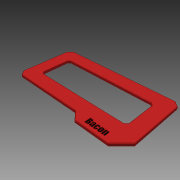
# Autodesk Inventor part: display_2004_frame
Saved by Autodesk Inventor 2014 (Build 180170000, 170)
## iProperties
Created: 2014-01-22
Part Number: display_2004_frame
Material: ABS Plastic
Document SubType Name: Modeling
Designer: buben
Density: 1.06 g/cm^3
Appearance: Light Red
Author: buben
Autodesk Inventor part; units mm, degrees
ref_plane "YZ Plane" through (0, 0, 0) normal (1, 0, 0) x (0, 1, 0)
ref_plane "XZ Plane" through (0, 0, 0) normal (0, 1, 0) x (-1, 0, 0)
ref_plane "XY Plane" through (0, 0, 0) normal (0, 0, 1) x (1, 0, 0)
sketch "Sketch1" plane through (0, 0, 0) normal (0, 1, 0) x (-1, 0, 0)
  line L0 (2, 0) -> (78, 0)
  line L1 (80, 2) -> (80, 25)
  line L2 (78, 27) -> (2, 27)
  line L3 (0, 25) -> (0, 2)
  line L4 (0, 25) -> (2, 27)
  line L5 (78, 27) -> (80, 25)
  line L6 (80, 2) -> (78, 0)
  line L7 (2, 0) -> (0, 2)
  line L8 (-8, 39) -> (88, 39)
  line L9 (92, 35) -> (92, -8)
  line L10 (88, -12) -> (-8, -12)
  line L11 (-12, -8) -> (-12, 35)
  line L12 (-12, 35) -> (-8, 39)
  line L13 (88, 39) -> (92, 35)
  line L14 (92, -8) -> (88, -12)
  line L15 (-8, -12) -> (-12, -8)
  point P0 (0, 0)
  point P1 (80, 27)
  point P2 (80, 0)
  point P3 (0, 27)
  point P4 (-12, 39)
  point P5 (92, -12)
  point P6 (92, 39)
  point P7 (-12, -12)
  point P8 (40, 39)
  point P9 (40, 27)
  point P10 (-12, 13.5)
  point P11 (0, 13.5)
  dimension "d0" = 2
  dimension "d1" = 2
  dimension "d2" = 2
  dimension "d3" = 2
  dimension "d4" = 2
  dimension "d5" = 2
  dimension "d6" = 2
  dimension "d7" = 2
  dimension "d8" = 80
  dimension "d9" = 27
  dimension "d10" = 4
  dimension "d11" = 4
  dimension "d12" = 4
  dimension "d13" = 4
  dimension "d14" = 4
  dimension "d15" = 4
  dimension "d16" = 4
  dimension "d17" = 4
  dimension "d18" = 12
  dimension "d19" = 12
  constraints: 32 end point, 16 point on line, 4 midpoint, 4 parallel, 2 horizontal, 2 perpendicular, 1 horizontal alignment, 1 vertical alignment
  measures "d0" distance of L3.start point (0, 27)
  measures "d1" distance of L2.end point (0, 27)
  measures "d2" distance of L2.start point (80, 27)
  measures "d3" distance of L1.end point (80, 27)
  measures "d4" distance of L1.start point (80, 0)
  measures "d5" distance of L0.end point (80, 0)
  measures "d6" distance of L0.start point (0, 0)
  measures "d7" distance of L3.end point (0, 0)
  measures "d8" distance between parallel lines of L1 L3
  measures "d9" distance between parallel lines of L0 L2
  measures "d10" distance of L11.end point (-12, 39)
  measures "d11" distance of L8.start point (-12, 39)
  measures "d12" distance of L8.end point (92, 39)
  measures "d13" distance of L9.start point (92, 39)
  measures "d14" distance of L9.end point (92, -12)
  measures "d15" distance of L10.start point (92, -12)
  measures "d16" distance of L10.end point (-12, -12)
  measures "d17" distance of L11.start point (-12, -12)
  measures "d18" distance between parallel lines of L3 L11
  measures "d19" distance between parallel lines of L2 L8
extrude "Extrusion1" add sketch "Sketch1" along normal blind 2
sketch "Sketch2" plane through (0, 2, 0) normal (0, 1, 0) x (1, 0, 0)
  line L0 (-92, -35) -> (-88, -39) projected
  line L1 (-88, -39) -> (8, -39) projected
  line L2 (8, -39) -> (2, -45)
  line L3 (2, -45) -> (-24, -45)
  line L4 (-24, -45) -> (-30, -39)
  point P0 (0, 0)
  dimension "d22" = 6
  dimension "d23" = 26
  constraints: 6 end point, 2 perpendicular, 1 parallel, 1 point on line
  measures "d22" distance between parallel lines of L1 L3
  measures "d23" distance of L2.end L3.end
extrude "Extrusion2" add sketch "Sketch2" against normal blind 2
chamfer "Chamfer1" distance 0.3 angle 45 18 edges at (-80, 2, 13.5) (-79, 2, 26) (-40, 2, 27) (-79, 2, 1) (-40, 2, 0) (-1, 2, 26) (0, 2, 13.5) (-1, 2, 1) (7, 2, 40) (12, 2, 13.5) (10, 2, -10) (-11, 2, 45) (-27, 2, 42) (-59, 2, 39) (-90, 2, 37) (-92, 2, 13.5) (-90, 2, -10) (-40, 2, -12)
sketch "Sketch3" plane through (0, 2, 0) normal (0, 1, 0) x (1, 0, 0)
  line L0 (-23.8757, -44.7) -> (-29.8757, -38.7) projected
  line L1 (1.8757, -44.7) -> (-23.8757, -44.7) projected
  line L2 (11.7, -34.8757) -> (1.8757, -44.7) projected
  line L3 (-29.8757, -38.7) -> (-87.8757, -38.7) projected
  line L4 (-21, -37.2) -> (-1, -37.2) construction
  line L5 (-1, -37.2) -> (-1, -42.2) construction
  line L6 (-1, -42.2) -> (-21, -42.2) construction
  line L7 (-21, -42.2) -> (-21, -37.2) construction
  line L8 (-21, -39.7) -> (-28.8757, -39.7) construction
  line L9 (-1, -39.7) -> (6.8757, -39.7) construction
  line L10 (-18.9145, -37.2) -> (-17.6183, -37.2)
  spline S0 degree 2 poles (-17.6183, -37.2) (-17.0004, -37.2) (-16.3674, -37.3922) (-15.9793, -37.9762) (-15.9793, -38.6243) knots 0 0 0 1 2 3 3 3
  spline S1 degree 2 poles (-15.9793, -38.6243) (-15.9793, -39.0613) (-16.2543, -39.408) (-16.6613, -39.4984) knots 0 0 0 1 2 2 2
  spline S2 degree 2 poles (-16.6613, -39.4984) (-16.2091, -39.6039) (-15.8888, -40.0749) (-15.8888, -40.5647) knots 0 0 0 1 2 2 2
  line L11 (-15.8888, -40.5647) -> (-15.8888, -41.0244)
  spline S3 degree 2 poles (-15.8888, -41.0244) (-15.8888, -41.5331) (-16.1187, -42.0191) (-16.6274, -42.2) (-17.4111, -42.2) knots 0 0 0 1 2 3 3 3
  line L12 (-17.4111, -42.2) -> (-18.9145, -42.2)
  line L13 (-18.9145, -42.2) -> (-18.9145, -37.2)
  line L14 (-17.6145, -39.9468) -> (-17.6145, -41.3447)
  spline S4 degree 2 poles (-17.6145, -41.3447) (-17.3395, -41.3372) (-17.1888, -41.1827) (-17.1888, -40.8775) knots 0 0 0 1 2 2 2
  line L15 (-17.1888, -40.8775) -> (-17.1888, -40.414)
  spline S5 degree 2 poles (-17.1888, -40.414) (-17.1888, -40.09) (-17.3244, -39.9543) (-17.6145, -39.9468) knots 0 0 0 1 2 2 2
  line L16 (-17.6145, -38.0553) -> (-17.6145, -39.1668)
  spline S6 degree 2 poles (-17.6145, -39.1668) (-17.5317, -39.1631) (-17.4864, -39.1631) knots 0 0 0 1 1 1
  spline S7 degree 2 poles (-17.4864, -39.1631) (-17.2943, -39.1631) (-17.1888, -38.9747) (-17.1888, -38.5301) knots 0 0 0 1 2 2 2
  spline S8 degree 2 poles (-17.1888, -38.5301) (-17.1888, -38.2965) (-17.2754, -38.1081) (-17.4148, -38.0591) (-17.6145, -38.0553) knots 0 0 0 1 2 3 3 3
  line L17 (-14.344, -39.6868) -> (-15.5158, -39.6868)
  line L18 (-15.5158, -39.6868) -> (-15.5158, -39.4118)
  spline S9 degree 2 poles (-15.5158, -39.4118) (-15.5158, -38.937) (-15.2973, -38.4208) (-14.6341, -38.0252) (-14.1066, -38.0252) knots 0 0 0 1 2 3 3 3
  spline S10 degree 2 poles (-14.1066, -38.0252) (-13.4736, -38.0252) (-12.8293, -38.4735) (-12.7012, -39.1254) (-12.7012, -40.1427) knots 0 0 0 1 2 3 3 3
  line L19 (-12.7012, -40.1427) -> (-12.7012, -42.2)
  line L20 (-12.7012, -42.2) -> (-13.9145, -42.2)
  line L21 (-13.9145, -42.2) -> (-13.9145, -41.8345)
  spline S11 degree 2 poles (-13.9145, -41.8345) (-14.0275, -42.0531) (-14.3892, -42.2754) (-14.6417, -42.2754) knots 0 0 0 1 2 2 2
  spline S12 degree 2 poles (-14.6417, -42.2754) (-14.9695, -42.2754) (-15.5158, -41.9061) (-15.5158, -41.2844) knots 0 0 0 1 2 2 2
  line L22 (-15.5158, -41.2844) -> (-15.5158, -40.9491)
  spline S13 degree 2 poles (-15.5158, -40.9491) (-15.5158, -40.4894) (-15.2257, -40.154) (-14.6492, -39.9317) knots 0 0 0 1 2 2 2
  spline S14 degree 2 poles (-14.6492, -39.9317) (-14.035, -39.6906) (-13.9484, -39.5248) (-13.9484, -39.2686) knots 0 0 0 1 2 2 2
  spline S15 degree 2 poles (-13.9484, -39.2686) (-13.9484, -38.9483) (-14.0426, -38.7524) (-14.1556, -38.7524) knots 0 0 0 1 2 2 2
  spline S16 degree 2 poles (-14.1556, -38.7524) (-14.2837, -38.7524) (-14.344, -38.9144) (-14.344, -39.2573) knots 0 0 0 1 2 2 2
  line L23 (-14.344, -39.2573) -> (-14.344, -39.6868)
  spline S17 degree 2 poles (-13.9484, -40.2482) (-14.2498, -40.4668) (-14.344, -40.7644) (-14.344, -41.0433) knots 0 0 0 1 2 2 2
  spline S18 degree 2 poles (-14.344, -41.0433) (-14.344, -41.3635) (-14.2611, -41.5482) (-14.1368, -41.5482) knots 0 0 0 1 2 2 2
  spline S19 degree 2 poles (-14.1368, -41.5482) (-14.02, -41.5482) (-13.9484, -41.4012) (-13.9484, -41.0922) knots 0 0 0 1 2 2 2
  line L24 (-13.9484, -41.0922) -> (-13.9484, -40.2482)
  line L25 (-9.5136, -39.6491) -> (-10.6891, -39.6491)
  line L26 (-10.6891, -39.6491) -> (-10.6891, -39.1744)
  spline S20 degree 2 poles (-10.6891, -39.1744) (-10.6891, -38.9295) (-10.7683, -38.7524) (-10.8775, -38.7524) knots 0 0 0 1 2 2 2
  spline S21 degree 2 poles (-10.8775, -38.7524) (-10.9868, -38.7524) (-11.0622, -38.9069) (-11.0622, -39.1744) knots 0 0 0 1 2 2 2
  line L27 (-11.0622, -39.1744) -> (-11.0622, -41.1111)
  spline S22 degree 2 poles (-11.0622, -41.1111) (-11.0622, -41.3296) (-10.9491, -41.5482) (-10.8436, -41.5482) knots 0 0 0 1 2 2 2
  spline S23 degree 2 poles (-10.8436, -41.5482) (-10.7155, -41.5482) (-10.6251, -41.3183) (-10.6251, -41.0018) knots 0 0 0 1 2 2 2
  line L28 (-10.6251, -41.0018) -> (-10.6251, -40.5157)
  line L29 (-10.6251, -40.5157) -> (-9.5136, -40.5157)
  spline S24 degree 2 poles (-9.5136, -40.5157) (-9.5173, -41.0056) (-9.5814, -41.4992) (-9.9318, -42.0116) (-10.4932, -42.2754) (-10.9077, -42.2754) knots 0 0 0 1 2 3 4 4 4
  spline S25 degree 2 poles (-10.9077, -42.2754) (-11.4352, -42.2754) (-12.0531, -41.9136) (-12.3093, -41.2618) (-12.3093, -40.6627) knots 0 0 0 1 2 3 3 3
  line L30 (-12.3093, -40.6627) -> (-12.3093, -39.4946)
  spline S26 degree 2 poles (-12.3093, -39.4946) (-12.3093, -38.9747) (-12.0983, -38.4434) (-11.4126, -38.0252) (-10.9228, -38.0252) knots 0 0 0 1 2 3 3 3
  spline S27 degree 2 poles (-10.9228, -38.0252) (-10.4329, -38.0252) (-9.7434, -38.4396) (-9.5136, -39.0689) (-9.5136, -39.6491) knots 0 0 0 1 2 3 3 3
  line L31 (-6.3222, -39.5399) -> (-6.3222, -40.5459)
  spline S28 degree 2 poles (-6.3222, -40.5459) (-6.3222, -41.096) (-6.4314, -41.6122) (-6.7969, -42.0606) (-7.3696, -42.2754) (-7.7389, -42.2754) knots 0 0 0 1 2 3 4 4 4
  spline S29 degree 2 poles (-7.7389, -42.2754) (-8.1534, -42.2754) (-8.7298, -42.0945) (-9.0463, -41.7252) (-9.182, -41.2015) (-9.182, -40.6815) knots 0 0 0 1 2 3 4 4 4
  line L32 (-9.182, -40.6815) -> (-9.182, -39.6303)
  spline S30 degree 2 poles (-9.182, -39.6303) (-9.182, -39.0576) (-8.9333, -38.4133) (-8.2928, -38.0252) (-7.7916, -38.0252) knots 0 0 0 1 2 3 3 3
  spline S31 degree 2 poles (-7.7916, -38.0252) (-7.3734, -38.0252) (-6.7705, -38.2739) (-6.4427, -38.677) (-6.3222, -39.1028) (-6.3222, -39.5399) knots 0 0 0 1 2 3 4 4 4
  spline S32 degree 2 poles (-7.5693, -39.2309) (-7.5693, -38.9144) (-7.6372, -38.7524) (-7.7502, -38.7524) knots 0 0 0 1 2 2 2
  spline S33 degree 2 poles (-7.7502, -38.7524) (-7.8595, -38.7524) (-7.9348, -38.9144) (-7.9348, -39.2309) knots 0 0 0 1 2 2 2
  line L33 (-7.9348, -39.2309) -> (-7.9348, -41.0809)
  spline S34 degree 2 poles (-7.9348, -41.0809) (-7.9348, -41.3711) (-7.8595, -41.5482) (-7.7502, -41.5482) knots 0 0 0 1 2 2 2
  spline S35 degree 2 poles (-7.7502, -41.5482) (-7.6409, -41.5482) (-7.5693, -41.3861) (-7.5693, -41.1224) knots 0 0 0 1 2 2 2
  line L34 (-7.5693, -41.1224) -> (-7.5693, -39.2309)
  line L35 (-4.6417, -38.1005) -> (-4.6643, -38.4773)
  spline S36 degree 2 poles (-4.6643, -38.4773) (-4.5286, -38.2512) (-4.1368, -38.0252) (-3.8806, -38.0252) knots 0 0 0 1 2 2 2
  spline S37 degree 2 poles (-3.8806, -38.0252) (-3.5565, -38.0252) (-3.1496, -38.3266) (-3.0328, -38.7901) (-3.0328, -39.3251) knots 0 0 0 1 2 3 3 3
  line L36 (-3.0328, -39.3251) -> (-3.0328, -42.2)
  line L37 (-3.0328, -42.2) -> (-4.28, -42.2)
  line L38 (-4.28, -42.2) -> (-4.28, -39.3628)
  spline S38 degree 2 poles (-4.28, -39.3628) (-4.28, -38.937) (-4.3365, -38.7524) (-4.4646, -38.7524) knots 0 0 0 1 2 2 2
  spline S39 degree 2 poles (-4.4646, -38.7524) (-4.5965, -38.7524) (-4.6643, -38.9671) (-4.6643, -39.4306) knots 0 0 0 1 2 2 2
  line L39 (-4.6643, -39.4306) -> (-4.6643, -42.2)
  line L40 (-4.6643, -42.2) -> (-5.9115, -42.2)
  line L41 (-5.9115, -42.2) -> (-5.9115, -38.1005)
  line L42 (-5.9115, -38.1005) -> (-4.6417, -38.1005)
  point P0 (0, 0)
  dimension "d29" = 20
  dimension "d30" = 5
  dimension "d31" = 6
  dimension "d32" = 5
  constraints: 4 end point, 3 collinear, 2 midpoint, 2 parallel, 2 point on line, 2 other
  measures "d29" distance of L4.start L4.end
  measures "d30" distance of L6.end L4.start
  measures "d31" distance between parallel lines of L3 L1
  measures "d32" distance between parallel lines of L1 L8
extrude "Extrusion3" cut sketch "Sketch3" against normal blind 0.3
equation "\"d1\" = d0"
equation "\"d2\" = d0"
equation "\"d3\" = d2"
equation "\"d4\" = d0"
equation "\"d5\" = d4"
equation "\"d6\" = d0"
equation "\"d7\" = d6"
equation "\"d11\" = d10"
equation "\"d12\" = d10"
equation "\"d13\" = d12"
equation "\"d14\" = d10"
equation "\"d15\" = d14"
equation "\"d16\" = d10"
equation "\"d17\" = d16"
equation "\"d19\" = d18"
body "Solid1"
